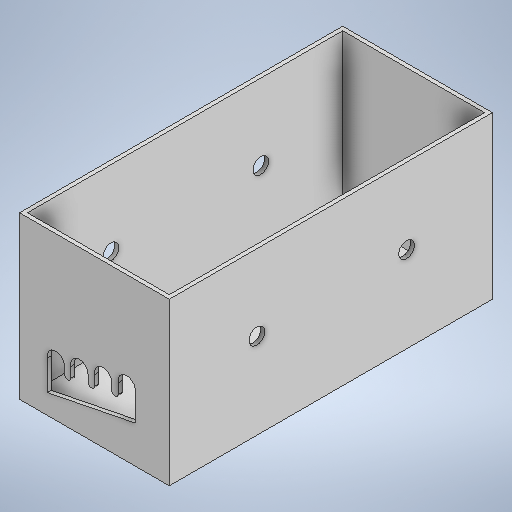
# Autodesk Inventor part: Box
Saved by Autodesk Inventor 2025.1 (Build 291241000, 241)
## iProperties
Created: 2024-11-05
Part Number: Box
Material: Generic
Document SubType Name: Modeling
Designer: Yash Purswani
Density: 1 g/cm^3
Appearance: Default
Author: Yash Purswani
Autodesk Inventor part; units mm, degrees
ref_plane "YZ Plane" through (0, 0, 0) normal (1, 0, 0) x (0, 1, 0)
ref_plane "XZ Plane" through (0, 0, 0) normal (0, 1, 0) x (-1, 0, 0)
ref_plane "XY Plane" through (0, 0, 0) normal (0, 0, 1) x (1, 0, 0)
sketch "Sketch1" plane through (0, 0, 0) normal (0, 1, 0) x (-1, 0, 0)
  line L0 (0, 0) -> (-90, 0)
  line L1 (-90, 0) -> (-90, -200)
  line L2 (-90, -200) -> (0, -200)
  line L3 (0, -200) -> (0, 0)
  line L4 (2.5, -202.5) -> (-92.5, -202.5)
  line L5 (-92.5, -202.5) -> (-92.5, 2.5)
  line L6 (-92.5, 2.5) -> (2.5, 2.5)
  line L7 (2.5, 2.5) -> (2.5, -202.5)
  line L8 (2.5, -202.5) -> (-92.5, 2.5) construction
  line L9 (-92.5, -202.5) -> (2.5, 2.5) construction
  point P0 (-45, -100)
  dimension "d0" = 90
  dimension "d1" = 200
  dimension "d2" = 95
  dimension "d3" = 205
  constraints: 20 end point, 4 parallel, 2 horizontal, 2 midpoint, 2 perpendicular
  measures "d0" distance of L2.end L1.end
  measures "d1" distance of L1.end L0.end
  measures "d2" distance of L5.end L6.end
  measures "d3" distance of L4.end L5.end
extrude "Extrusion1" add sketch "Sketch1" along normal blind 100
sketch "Sketch2" plane through (0, 0, 0) normal (0, -1, 0) x (1, 0, 0)
  line L0 (92.5, 2.5) -> (-2.5, 2.5)
  line L1 (-2.5, 2.5) -> (-2.5, -202.5)
  line L2 (-2.5, -202.5) -> (92.5, -202.5)
  line L3 (92.5, -202.5) -> (92.5, 2.5)
  point P0 (0, 0)
  constraints: 8 end point, 2 parallel, 1 horizontal, 1 perpendicular
extrude "Extrusion2" add sketch "Sketch2" along normal blind 2.5
sketch "Sketch3" plane through (-2.5, 100, 2.5) normal (0, 0, 1) x (1, 0, 0)
  line L0 (2.5, -100) -> (17.5, -100)
  line L1 (92.5, -100) -> (2.5, -100) projected
  line L2 (17.5, -100) -> (17.5, -90)
  line L3 (17.5, -90) -> (77.5, -90)
  line L4 (77.5, -90) -> (77.5, -78)
  line L5 (77.5, -78) -> (17.5, -90)
  line L6 (17.5, -90) -> (17.5, -80)
  line L7 (17.5, -80) -> (17.5, -70)
  line L8 (17.5, -70) -> (23, -70)
  circle A0 centre (23, -70) radius 5.5
  line L9 (28.5, -70) -> (28.5, -76.5)
  line L10 (96.033, -55.3934) -> (23, -70)
  line L11 (17.6068, -71.0786) -> (17.5, -71.1)
  line L12 (23, -70) -> (38, -70)
  line L13 (38, -70) -> (38, -67)
  circle A1 centre (38, -67) radius 5.5
  line L14 (38, -67) -> (53, -67)
  line L15 (53, -67) -> (53, -64)
  line L16 (53, -64) -> (68, -64)
  line L17 (68, -64) -> (68, -61)
  circle A2 centre (53, -64) radius 5.5
  circle A3 centre (68, -61) radius 5.5
  line L18 (32.6068, -68.0786) -> (32.6068, -76.5)
  line L19 (43.5, -67) -> (43.5, -73.5)
  line L20 (47.6068, -65.0786) -> (47.6068, -73.5)
  line L21 (58.5, -64) -> (58.5, -70.5)
  line L22 (62.6068, -62.0786) -> (62.6068, -70.5)
  line L23 (73.3932, -59.9214) -> (73.3932, -78.8214)
  line L24 (28.5, -76.5) -> (32.6068, -76.5)
  line L25 (43.5, -73.5) -> (47.6068, -73.5)
  line L26 (58.5, -70.5) -> (62.6068, -70.5)
  circle A4 centre (30.5534, -74.4466) radius 2.0534
  circle A5 centre (45.5534, -71.4466) radius 2.0534
  circle A6 centre (60.5534, -68.4466) radius 2.0534
  point P0 (32.6068, -74.4466)
  point P1 (28.5, -74.4466)
  point P2 (62.6068, -68.4466)
  point P3 (58.5, -68.4466)
  point P4 (47.6068, -71.4466)
  point P5 (43.5, -71.4466)
  dimension "d9" = 15
  dimension "d10" = 10
  dimension "d11" = 90
  dimension "d12" = 60
  dimension "d13" = 12
  dimension "d14" = 10
  dimension "d15" = 10
  dimension "d16" = 5.5
  dimension "d17" = 6.5
  dimension "d18" = 15
  dimension "d19" = 11
  dimension "d20" = 15
  dimension "d21" = 15
  dimension "d22" = 11
  dimension "d23" = 11
  dimension "d24" = 6.5
  dimension "d25" = 6.5
  constraints: 50 end point, 12 tangent, 11 perpendicular, 9 point on circle, 7 centre point, 6 vertical, 5 point on line, 4 coincident, 4 horizontal, 1 parallel, 10 other
  measures "d9" distance of L0.start L0.end
  measures "d10" distance of L0.end L2.end
  measures "d11" angle of L2 L0
  measures "d12" distance of L2.end L3.end
  measures "d13" distance of L3.end L4.end
  measures "d14" distance of L2.end L6.end
  measures "d15" distance of L6.end L7.end
  measures "d16" distance of L7.end L8.end
  measures "d17" distance of L9.start L9.end
  measures "d18" distance of L12.start L12.end
  measures "d19" diameter of A1
  measures "d20" distance of L14.start L14.end
  measures "d21" distance of L15.end L16.end
  measures "d22" diameter of A2
  measures "d23" diameter of A3
  measures "d24" distance of L19.start L19.end
  measures "d25" distance of L21.start L21.end
extrude "Extrusion3" cut sketch "Sketch3" against normal blind 15 contours L6 L7 L11 A0 L9 L24 L18 L12 A1 L19 L25 L20 L14 A2 L21 L26 L22 L16 A3 L23 L5 | A3 L16 L17 L10 L23 | A3 L10 L17 L16 | L16 L22 A3 | L10 A3 | A0 L10 L8 | L8 L12 A0 | L10 A0 L12 | A2 L14 L15 L16 | L16 L10 A2 | L22 L26 A6 | L10 A2 | A1 L10 | L10 L13 L12 A1 | A1 L12 L18 | A4 L24 L9 | L15 L14 A2 L10 | L14 L20 A2 | A6 L26 L21 | L14 A1 L12 L13 | L10 A1 L14 | L18 L24 A4 | L20 L25 A5 | A5 L25 L19
sketch "Sketch4" plane through (-2.5, 100, -202.5) normal (-1, 0, 0) x (0, 0, 1)
  line L0 (202.5, -100) -> (2.5, -100) projected
  line L1 (2.5, -100) -> (2.5, -90)
  line L2 (2.5, -100) -> (2.5, 0) projected
  line L3 (2.5, -90) -> (54.5, -90)
  line L4 (54.5, -90) -> (54.5, -48)
  circle A0 centre (54.5, -48) radius 5
  line L5 (54.5, -48) -> (149.5, -48)
  circle A1 centre (149.5, -48) radius 5
  dimension "d28" = 10
  dimension "d29" = 52
  dimension "d30" = 42
  dimension "d31" = 10
  dimension "d32" = 95
  dimension "d33" = 10
  constraints: 8 end point, 2 centre point, 2 coincident, 2 perpendicular, 1 horizontal, 1 point on line
  measures "d28" distance of L0.end L1.end
  measures "d29" distance of L1.end L3.end
  measures "d30" distance of L3.end L4.end
  measures "d31" diameter of A0
  measures "d32" distance of L5.start L5.end
  measures "d33" diameter of A1
extrude "Extrusion4" cut sketch "Sketch4" against normal through all
equation "\"d26\" = d20"
body "Solid1"
